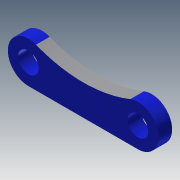
# Autodesk Inventor part: tahlo5(b)
Saved by Autodesk Inventor 2013 (Build 170138000, 138)
## iProperties
Created: 2013-02-02
Part Number: tahlo5(b)
Material: Generic
Document SubType Name: Modeling
Designer: idle-rug
Density: 1 g/cm^3
Author: idle-rug
Autodesk Inventor part; units mm, degrees
ref_plane "YZ Plane" through (0, 0, 0) normal (1, 0, 0) x (0, 1, 0)
ref_plane "XZ Plane" through (0, 0, 0) normal (0, 1, 0) x (-1, 0, 0)
ref_plane "XY Plane" through (0, 0, 0) normal (0, 0, 1) x (1, 0, 0)
sketch "Sketch1" plane through (0, 0, 0) normal (0, 1, 0) x (-1, 0, 0)
  line L0 (-8, -3) -> (8, -3)
  line L1 (8, -3) -> (8, 3)
  line L2 (8, 3) -> (-8, 3)
  line L3 (-8, 3) -> (-8, -3)
  line L4 (-8, -3) -> (8, 3) construction
  line L5 (8, -3) -> (-8, 3) construction
  circle A0 centre (8, 0) radius 3
  circle A1 centre (-8, 0) radius 3
  point P0 (0, 0)
  dimension "d0" = 16
  dimension "d1" = 6
  dimension "d2" = 6
  dimension "d3" = 6
  constraints: 12 end point, 4 midpoint, 2 centre point, 2 parallel, 1 horizontal, 1 perpendicular
  measures "d0" distance of L2.end L1.end
  measures "d1" distance of L1.end L0.end
  measures "d2" diameter of A0
  measures "d3" diameter of A1
extrude "Extrusion1" add sketch "Sketch1" along normal blind 2
sketch "Sketch2" plane through (0, 2, 0) normal (0, 1, 0) x (1, 0, 0)
  arc A0 (8, -3) -> (8, 3) centre (8, 0) ccw projected
  arc A1 (-8, 3) -> (-8, -3) centre (-8, 0) ccw projected
  circle A2 centre (-8, 0) radius 1.5
  circle A3 centre (8, 0) radius 1.5
  point P0 (0, 0)
  dimension "d6" = 3
  dimension "d7" = 3
  constraints: 2 centre point, 2 coincident
  measures "d6" diameter of A2
  measures "d7" diameter of A3
extrude "Extrusion2" cut sketch "Sketch2" against normal blind 2
sketch "Sketch3" plane through (0, 0, 0) normal (0, -1, 0) x (1, 0, 0)
  line L0 (-8, 3) -> (8, 3) projected
  line L1 (0, 0) -> (0, 20)
  circle A0 centre (0, 20) radius 18.5407
  dimension "d11" = 20
  constraints: 2 end point, 1 centre point, 1 coincident, 1 perpendicular
  measures "d11" distance of L1.start L1.end
extrude "Extrusion3" cut sketch "Sketch3" against normal blind 2
sketch "Sketch4" plane through (0, 0, 0) normal (0, -1, 0) x (1, 0, 0)
  arc A0 (-7.3997, 3) -> (7.3997, 3) centre (0, 20) ccw projected
  circle A1 centre (-8, 0) radius 1.5 projected
  circle A2 centre (8, 0) radius 1.5 projected
  circle A3 centre (-8, 0) radius 3
  circle A4 centre (8, 0) radius 3
  point P0 (0, 0)
  constraints: 2 centre point, 2 coincident, 2 tangent
extrude "Extrusion4" cut sketch "Sketch4" against normal blind 2
sketch "Sketch5" plane through (0, 0, 0) normal (0, -1, 0) x (1, 0, 0)
  arc A0 (8, 3) -> (6.8858, 2.7854) centre (8, 0) ccw projected
  line L0 (7.3997, 3) -> (8, 3) projected
  arc A1 (6.8858, 2.7854) -> (7.3997, 3) centre (0, 20) ccw projected
  point P0 (0, 0)
extrude "Extrusion5" cut sketch "Sketch5" against normal blind 2
sketch "Sketch6" plane through (0, 0, 0) normal (0, -1, 0) x (1, 0, 0)
  arc A0 (-6.8858, 2.7854) -> (-8, 3) centre (-8, 0) ccw projected
  arc A1 (-7.3997, 3) -> (-6.8858, 2.7854) centre (0, 20) ccw projected
  line L0 (-8, 3) -> (-7.3997, 3) projected
  point P0 (0, 0)
extrude "Extrusion6" cut sketch "Sketch6" against normal blind 2
sketch "Sketch7" plane through (0, 0, 0) normal (0, -1, 0) x (1, 0, 0)
  arc A0 (-8, -3) -> (-6.8858, 2.7854) centre (-8, 0) ccw projected
  arc A1 (6.8858, 2.7854) -> (8, -3) centre (8, 0) ccw projected
  circle A2 centre (-8, 0) radius 3
  circle A3 centre (8, 0) radius 3
  circle A4 centre (-8, 0) radius 3
  circle A5 centre (-8, 0) radius 1.5
  circle A6 centre (8, 0) radius 1.5
  point P0 (0, 0)
  dimension "d20" = 6
  dimension "d21" = 3
  dimension "d22" = 3
  constraints: 5 coincident, 4 centre point, 1 concentric, 1 vertical alignment, 2 other
  measures "d20" diameter of A4
  measures "d21" diameter of A5
  measures "d22" diameter of A6
extrude "Extrusion7" add sketch "Sketch7" against normal blind 2
body "Solid1"
